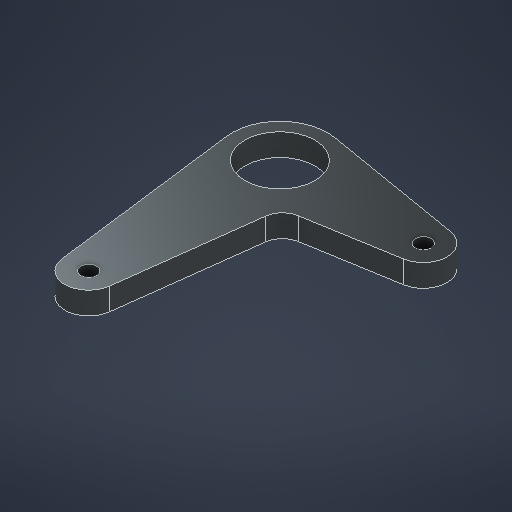
# Autodesk Inventor part: BellCrank
Saved by Autodesk Inventor 2026.2 (Build 302298010, 298A)
## iProperties
Created: 2026-07-07
Part Number: BellCrank
Material: Generic
Document SubType Name: Modeling
Designer: tasle
Density: 1 g/cm^3
Appearance: Iron Gray
Author: tasle
Autodesk Inventor part; units mm, degrees
ref_plane "YZ Plane" through (0, 0, 0) normal (1, 0, 0) x (0, 1, 0)
ref_plane "XZ Plane" through (0, 0, 0) normal (0, 1, 0) x (-1, 0, 0)
ref_plane "XY Plane" through (0, 0, 0) normal (0, 0, 1) x (1, 0, 0)
sketch "Sketch1" plane through (0, 0, 0) normal (0, 1, 0) x (-1, 0, 0)
  circle A0 centre (0, 0) radius 11
  circle A1 centre (0, 0) radius 15
  circle A2 centre (0, 60) radius 7.5
  circle A3 centre (-45, 0) radius 7.5
  line L0 (0, 60) -> (0, 0)
  line L1 (0, 0) -> (-45, 0)
  line L2 (7.4412, 60.9375) -> (14.8824, 1.875)
  line L3 (-14.8824, 1.875) -> (-7.4412, 60.9375)
  line L4 (-2.5, 14.7902) -> (-46.25, 7.3951)
  line L5 (-2.5, -14.7902) -> (-46.25, -7.3951)
  circle A4 centre (0, 60) radius 2.5
  circle A5 centre (-45, 0) radius 2.5
  point P0 (-13.4892, 12.9327)
  dimension "d0" = 22
  dimension "d1" = 30
  dimension "d2" = 15
  dimension "d3" = 15
  dimension "d4" = 45
  dimension "d5" = 60
  dimension "d6" = 5
  dimension "d7" = 5
  constraints: 12 end point, 8 point on circle, 8 tangent, 6 centre point, 4 coincident, 1 perpendicular, 1 vertical
  measures "d0" diameter of A0
  measures "d1" diameter of A1
  measures "d2" diameter of A2
  measures "d3" diameter of A3
  measures "d4" distance of L0.end L1.end
  measures "d5" distance of L0.start L0.end
  measures "d6" diameter of A4
  measures "d7" diameter of A5
extrude "Extrusion1" add sketch "Sketch1" along normal blind 7 contours A0 L0 A1 L1 | A0 L1 A1 L0 | L0 A2 L2 A1 | A1 L4 L3 A2 L0 | L1 A3 L4 L3 A1 | A1 L5 A3 L1 | A1 L3 L4 | A2 | A3
fillet "Fillet1" radius 6 1 edges at (13.4892, 3.5, 12.9327)
body "Solid1"
